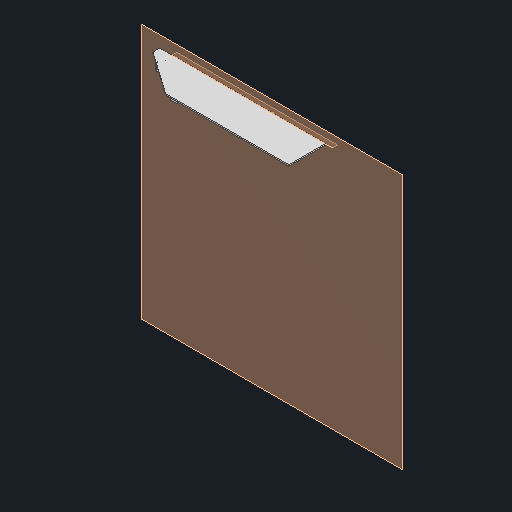
# Autodesk Inventor part: right_side
Saved by Autodesk Inventor 2023 (Build 270158000, 158)
## iProperties
Created: 2024-05-19
Part Number: right_side
Material: Generic
Document SubType Name: Modeling
Designer: szymo
Density: 1 g/cm^3
Appearance: Default
Mass: 4.02235 g
Surface Area: 72.4385 cm^2
Volume: 4.02235 cm^3
Author: szymo
Autodesk Inventor part; units mm, degrees
ref_plane "YZ Plane" through (0, 0, 0) normal (1, 0, 0) x (0, 1, 0)
ref_plane "XZ Plane" through (0, 0, 0) normal (0, 1, 0) x (-1, 0, 0)
ref_plane "XY Plane" through (0, 0, 0) normal (0, 0, 1) x (1, 0, 0)
ref_plane "Work Plane1" through (41, 89, -3.5) normal (0, 1, 0) x (-1, 0, 0)
sketch "Sketch1" plane through (41, 89, -3.5) normal (0, 1, 0) x (-1, 0, 0)
  arc A0 (0, 27.0092) -> (4.4908, 31.5) centre (3, 28.5) ccw projected
  line L0 (0, 3.5) -> (0, 27.0092) projected
  line L1 (0, 3.5) -> (99.4519, 3.5) projected
  line L2 (99.4519, 3.5) -> (97.9046, 17.0805) projected
  line L3 (97.9046, 17.0805) -> (86.1669, 8.8617) projected
  line L4 (85.0198, 8.5) -> (76.1137, 8.5) projected
  line L5 (74.9666, 12.1383) -> (92.1507, 24.1708) projected
  line L6 (94.445, 24.1708) -> (98.8981, 21.0527) projected
  line L7 (99.5829, 18.612) -> (109.4208, 19.7329) projected
  line L8 (109.4208, 19.7329) -> (111.1189, 4.8293) projected
  line L9 (111.1189, 4.8293) -> (99.4519, 3.5) projected
  line L10 (99.4519, 3.5) -> (127, 3.5) projected
  line L11 (127, 3.5) -> (127, 8.7002) projected
  line L12 (127, 8.7002) -> (123.75, 8.7002) projected
  line L13 (123.75, 8.7002) -> (120.5, 8.7002) projected
  arc A1 (116.1068, 16.3277) -> (120.5, 8.7002) centre (127.9773, 18.0858) ccw projected
  line L14 (116.1068, 16.3277) -> (94.4385, 31.5) projected
  line L15 (94.4385, 31.5) -> (27.4908, 31.5) projected
  arc A2 (24.5092, 31.5) -> (27.4908, 31.5) centre (26, 28.5) ccw projected
  line L16 (24.5092, 31.5) -> (4.4908, 31.5) projected
  circle A3 centre (15.5, 17.5) radius 5 projected
  arc A4 (6.5587, 12.2463) -> (10.9717, 8.1704) centre (15.5, 17.5) ccw projected
  arc A5 (7.2428, 14.3769) -> (6.5587, 12.2463) centre (7.852, 13.0062) ccw projected
  line L17 (7.2428, 14.3769) -> (8.2553, 14.827) projected
  arc A6 (10.1455, 14.2369) -> (8.2553, 14.827) centre (8.8646, 13.4563) ccw projected
  arc A7 (10.1455, 14.2369) -> (12.6717, 11.9036) centre (15.5, 17.5) ccw projected
  arc A8 (13.4098, 10.0662) -> (12.6717, 11.9036) centre (11.9951, 10.5649) ccw projected
  line L18 (13.4098, 10.0662) -> (13.0414, 9.0211) projected
  arc A9 (10.9717, 8.1704) -> (13.0414, 9.0211) centre (11.6267, 9.5198) ccw projected
  arc A10 (20.0283, 26.8296) -> (17.9586, 25.9789) centre (19.3733, 25.4802) ccw projected
  arc A11 (24.4413, 22.7537) -> (20.0283, 26.8296) centre (15.5, 17.5) ccw projected
  arc A12 (23.7572, 20.6231) -> (24.4413, 22.7537) centre (23.148, 21.9938) ccw projected
  line L19 (23.7572, 20.6231) -> (22.7447, 20.173) projected
  arc A13 (20.8545, 20.7631) -> (22.7447, 20.173) centre (22.1354, 21.5437) ccw projected
  arc A14 (20.8545, 20.7631) -> (18.3283, 23.0964) centre (15.5, 17.5) ccw projected
  arc A15 (17.5902, 24.9338) -> (18.3283, 23.0964) centre (19.0049, 24.4351) ccw projected
  line L20 (17.5902, 24.9338) -> (17.9586, 25.9789) projected
  arc A16 (6.5587, 22.7537) -> (7.2428, 20.6231) centre (7.852, 21.9938) ccw projected
  arc A17 (10.9717, 26.8296) -> (6.5587, 22.7537) centre (15.5, 17.5) ccw projected
  arc A18 (13.0414, 25.9789) -> (10.9717, 26.8296) centre (11.6267, 25.4802) ccw projected
  line L21 (13.0414, 25.9789) -> (13.4098, 24.9338) projected
  arc A19 (12.6717, 23.0964) -> (13.4098, 24.9338) centre (11.9951, 24.4351) ccw projected
  arc A20 (8.2553, 20.173) -> (10.1455, 20.7631) centre (8.8646, 21.5437) ccw projected
  line L22 (8.2553, 20.173) -> (7.2428, 20.6231) projected
  arc A21 (20.0283, 8.1704) -> (24.4413, 12.2463) centre (15.5, 17.5) ccw projected
  arc A22 (17.9586, 9.0211) -> (20.0283, 8.1704) centre (19.3733, 9.5198) ccw projected
  line L23 (17.9586, 9.0211) -> (17.5902, 10.0662) projected
  arc A23 (18.3283, 11.9036) -> (17.5902, 10.0662) centre (19.0049, 10.5649) ccw projected
  arc A24 (18.3283, 11.9036) -> (20.8545, 14.2369) centre (15.5, 17.5) ccw projected
  arc A25 (22.7447, 14.827) -> (20.8545, 14.2369) centre (22.1354, 13.4563) ccw projected
  line L24 (22.7447, 14.827) -> (23.7572, 14.3769) projected
  arc A26 (24.4413, 12.2463) -> (23.7572, 14.3769) centre (23.148, 13.0062) ccw projected
  line L25 (60.4227, 8.5) -> (45.5604, 8.5) projected
  line L26 (44.4133, 12.1383) -> (64.4073, 26.1383) projected
  line L27 (65.5545, 26.5) -> (80.4168, 26.5) projected
  line L28 (81.5639, 22.8617) -> (61.5699, 8.8617) projected
  line L29 (30.5, 12.342) -> (30.5, 26.5) projected
  line L30 (32.5, 28.5) -> (52.7198, 28.5) projected
  line L31 (53.8669, 24.8617) -> (33.6472, 10.7037) projected
  line L32 (0, 3.5) -> (94.4385, 3.5)
  line L33 (94.4385, 3.5) -> (94.4385, 31.5)
  line L34 (94.4385, 31.5) -> (0, 31.5)
  line L35 (0, 31.5) -> (0, 3.5)
  line L36 (94.4385, 31.5) -> (127, 8.7002)
  line L37 (127, 8.7002) -> (127, 3.5)
  line L38 (127, 3.5) -> (94.4385, 3.5)
  arc A27 (12.6717, 23.0964) -> (10.1455, 20.7631) centre (15.5, 17.5) ccw projected
  arc A28 (85.0198, 8.5) -> (86.1669, 8.8617) centre (85.0198, 10.5) ccw projected
  arc A29 (74.9666, 12.1383) -> (76.1137, 8.5) centre (76.1137, 10.5) ccw projected
  arc A30 (94.445, 24.1708) -> (92.1507, 24.1708) centre (93.2979, 22.5325) ccw projected
  arc A31 (99.5829, 18.612) -> (98.8981, 21.0527) centre (97.7509, 19.4144) ccw projected
  circle A32 centre (15.5, 25.5) radius 1.8 projected
  circle A33 centre (15.5, 9.5) radius 1.8 projected
  arc A34 (44.4133, 12.1383) -> (45.5604, 8.5) centre (45.5604, 10.5) ccw projected
  arc A35 (65.5545, 26.5) -> (64.4073, 26.1383) centre (65.5545, 24.5) ccw projected
  arc A36 (81.5639, 22.8617) -> (80.4168, 26.5) centre (80.4168, 24.5) ccw projected
  arc A37 (60.4227, 8.5) -> (61.5699, 8.8617) centre (60.4227, 10.5) ccw projected
  arc A38 (32.5, 28.5) -> (30.5, 26.5) centre (32.5, 26.5) ccw projected
  arc A39 (53.8669, 24.8617) -> (52.7198, 28.5) centre (52.7198, 26.5) ccw projected
  arc A40 (30.5, 12.342) -> (33.6472, 10.7037) centre (32.5, 12.342) ccw projected
  point P0 (41, 3.5)
  point P1 (27.4908, 31.5)
  point P2 (24.5092, 31.5)
  point P3 (4.4908, 31.5)
  point P4 (0, 27.0092)
  constraints: 14 end point, 3 equal length, 2 perpendicular, 1 horizontal
extrude "Extrusion1" add sketch "Sketch1" against normal blind 1 contours L35 L34 A0 | A0 L16 A2 L15 L33 A30 L5 A29 L4 A28 L3 L1 L0 | L34 A2 | L33 L3 L2 L1 | L2 L3 L33 A30 L6 A31 L7 L8 L9 | L9 L8 L7 A31 L6 A30 L33 L14 A1 L13 L12 L11 L10 | L3 A28 L4 A29 L5 A30 L33 | L36 L12 L13 A1 | A3 | A5 L17 A6 A7 A8 L18 A9 A4 | A11 A12 L19 A13 A14 A15 L20 A10 | A17 A18 L21 A19 A27 A20 L22 A16 | A22 L23 A23 A24 A25 L24 A26 A21 | L25 A34 L26 A35 L27 A36 L28 A37 | L29 A38 L30 A39 L31 A40 | A32 | A33
sketch "Sketch2" plane through (41, 88, -3.5) normal (0, -1, 0) x (1, 0, 0)
  point P0 (-41, 3.5)
sketch "Sketch3" plane through (41, 88, -3.5) normal (0, -1, 0) x (1, 0, 0)
  line L0 (-127, 3.5) -> (0, 3.5) projected
  line L1 (0, 3.5) -> (0, 31.5) projected
  line L2 (0, 31.5) -> (-94.4385, 31.5) projected
  line L3 (-94.4385, 31.5) -> (-127, 8.7002) projected
  line L4 (-127, 8.7002) -> (-127, 3.5) projected
  line L5 (-118.25, 3.5) -> (-115.75, 3.5) projected
  line L6 (-118.25, 3.5) -> (-115.75, 3.5)
  line L7 (-115.75, 3.5) -> (-115.75, 7)
  line L8 (-115.75, 7) -> (-118.25, 7)
  line L9 (-118.25, 7) -> (-118.25, 3.5)
  line L10 (-123.5, 5.5) -> (-123.5, 3.5) projected
  line L11 (-121.5, 3.5) -> (-112, 3.5)
  line L12 (-112, 3.5) -> (-112, 19.2033)
  line L13 (-112, 19.2033) -> (-121.5, 19.2033)
  line L14 (-121.5, 19.2033) -> (-121.5, 3.5)
  line L15 (-112.5, 3.5) -> (-126.5, 3.5) projected
  line L16 (-112, 3.5) -> (-128, 3.5) projected
  line L17 (-121.5, 3.5) -> (-112, 3.5)
  line L18 (-112, 3.5) -> (-112, 8.5)
  line L19 (-112, 8.5) -> (-121.5, 8.5)
  line L20 (-121.5, 8.5) -> (-121.5, 3.5)
  point P0 (-41, 3.5)
  dimension "d2" = 3.5
  dimension "d3" = 2
  dimension "d5" = 5
  constraints: 24 end point, 6 parallel, 4 point on line, 3 horizontal, 3 perpendicular, 1 other
  measures "d2" distance of L7.end L6.end
  measures "d3" distance from line of L14 L10.start
  measures "d5" distance between parallel lines of L19 L15
extrude "Extrusion2" add sketch "Sketch3" along normal blind 12 contours L14 L19 L12 L0 L7 L8 L9 | L9 L8 L7 L0
sketch "Sketch4" plane through (41, 88, -3.5) normal (0, -1, 0) x (1, 0, 0)
  line L0 (-121.5, 3.5) -> (-121.5, 8.5) projected
  line L1 (-121.5, 8.5) -> (-112, 8.5) projected
  line L2 (-112, 8.5) -> (-112, 3.5) projected
  line L3 (-112, 3.5) -> (0, 3.5) projected
  line L4 (0, 3.5) -> (0, 31.5) projected
  line L5 (0, 31.5) -> (-94.4385, 31.5) projected
  line L6 (-94.4385, 31.5) -> (-127, 8.7002) projected
  line L7 (-127, 8.7002) -> (-127, 3.5) projected
  line L8 (-127, 3.5) -> (-121.5, 3.5) projected
  line L9 (-121.4366, 12.5958) -> (-117.3408, 15.4636)
  line L10 (-117.3408, 15.4636) -> (-114.4729, 11.3679)
  line L11 (-114.4729, 11.3679) -> (-118.5687, 8.5)
  line L12 (-118.5687, 8.5) -> (-121.4366, 12.5958)
  line L13 (-112, 8.5) -> (-121.5, 8.5) projected
  line L14 (-121.4366, 12.5958) -> (-121.5, 8.5)
  line L15 (-114.4729, 11.3679) -> (-112, 8.5)
  point P0 (-41, 3.5)
  dimension "d8" = 5
  dimension "d9" = 5
  constraints: 12 end point, 3 point on line, 2 parallel, 1 perpendicular
  measures "d8" distance of L9.start L9.end
  measures "d9" distance of L9.end L10.end
extrude "Extrusion3" add sketch "Sketch4" along normal blind 4 contours L14 L12 L1 | L11 L15 L1 | L12 L6 L10 L11
sketch "Sketch5" plane through (-86, 88, 5.2002) normal (-0.5735764, 0, 0.819152) x (0.819152, 0, 0.5735764)
  line L0 (0, 1) -> (39.7502, 1) projected
  line L1 (0, 1) -> (0, 0) projected
  line L2 (6.7917, 0) -> (0, 0) projected
  line L3 (6.7917, 0) -> (6.7917, -4) projected
  line L4 (11.7917, -4) -> (6.7917, -4) projected
  line L5 (11.7917, 0) -> (11.7917, -4) projected
  line L6 (39.7502, 0) -> (11.7917, 0) projected
  line L7 (39.7502, 1) -> (39.7502, 0) projected
  line L8 (6.7917, -4) -> (11.7917, -4)
  line L9 (11.7917, -4) -> (11.7917, 1)
  line L10 (11.7917, 1) -> (6.7917, 1)
  line L11 (6.7917, 1) -> (6.7917, -4)
  line L12 (11.7917, -4) -> (6.7917, 1)
  line L13 (6.7917, -4) -> (11.7917, 1)
  line L14 (9.3046, 0) -> (9.3046, -12) projected
  point P0 (67.4644, -88)
  point P1 (9.3046, -1.4871)
  constraints: 12 end point, 3 point on line, 2 parallel, 2 perpendicular, 1 horizontal
hole "Hole1" at (-78.3781, 86.5129, 10.5371) direction (0.5735764, 0, -0.819152) diameter 4 depth 5.5 counterbore diameter 4.6 counterbore depth 1
ref_plane "Work Plane2" through (0, 0, 0) normal (0, 0, 1) x (1, 0, 0)
sketch "Sketch6" plane through (0, 0, 0) normal (0, 0, 1) x (1, 0, 0)
  ellipse E0 centre (-78.3781, 86.5129) end of major axis (-78.3781, 84.2129) minor radius 1.884 projected
  line L0 (-86, 89) -> (-53.4385, 89) projected
  line L1 (-86, 89) -> (-86, 88) projected
  line L2 (-80.4366, 88) -> (-86, 88) projected
  line L3 (-80.4366, 88) -> (-80.4366, 84) projected
  line L4 (-76.3408, 84) -> (-80.4366, 84) projected
  line L5 (-76.3408, 88) -> (-76.3408, 84) projected
  line L6 (-53.4385, 88) -> (-76.3408, 88) projected
  line L7 (-53.4385, 89) -> (-53.4385, 88) projected
  line L8 (-73.4729, 88) -> (-71, 88) projected
  line L9 (-73.4729, 88) -> (-73.4729, 84) projected
  line L10 (-71, 84) -> (-73.4729, 84) projected
  line L11 (-71, 88) -> (-71, 84) projected
  line L12 (-71, 84) -> (-80.5, 84) projected
  line L13 (-80.5, 84) -> (-80.5, 76) projected
  line L14 (-71, 76) -> (-80.5, 76) projected
  line L15 (-71, 84) -> (-71, 76) projected
  line L16 (-71, 88) -> (-71, 76) projected
  line L17 (-71, 88) -> (-64, 88)
  line L18 (-64, 88) -> (-64, 81)
  line L19 (-64, 81) -> (-71, 81)
  line L20 (-71, 81) -> (-71, 88)
  point P0 (0, 0)
  dimension "d19" = 7
  dimension "d20" = 7
  constraints: 8 end point, 2 parallel, 1 horizontal, 1 perpendicular, 1 other
  measures "d19" distance of L18.end L19.end
  measures "d20" distance of L17.end L18.end
extrude "Extrusion4" add sketch "Sketch6" along normal up to surface (5 mm away) contours L18 L19 L15 L11 L6
sketch "Sketch7" plane through (-80.5, 76, 5) normal (0, 0, 1) x (1, 0, 0)
  line L0 (9.5, 8) -> (0, 8) projected
  line L1 (0, 8) -> (0, 0) projected
  line L2 (9.5, 0) -> (0, 0) projected
  line L3 (9.5, 5) -> (9.5, 0) projected
  line L4 (16.5, 5) -> (9.5, 5) projected
  line L5 (16.5, 12) -> (16.5, 5) projected
  line L6 (9.5, 12) -> (16.5, 12) projected
  line L7 (9.5, 12) -> (9.5, 8) projected
  line L8 (16.5, 5) -> (9.5, 12)
  point P0 (80.5, -76)
  point P1 (13, 8.5)
  constraints: 2 end point, 1 midpoint
hole "Hole2" at (-67.5, 84.5, 5) direction (0, 0, -1) diameter 3.6 end through all countersink diameter 6.5 countersink angle 90 clearance for "Countersunk Flat Head Screw ISO 2009/7046" size "M3" standard "ISO"
ref_plane "Work Plane3" through (0, 0, 0) normal (0, 0, 1) x (1, 0, 0)
sketch "Sketch9" plane through (-71, 81, 0) normal (0, -1, 0) x (1, 0, 0)
  line L0 (7, 5) -> (0, 5) projected
  line L1 (0, 0) -> (0, 5) projected
  line L2 (0, 0) -> (7, 0) projected
  line L3 (7, 0) -> (7, 5) projected
  line L4 (0, 5) -> (7, 5) projected
  line L5 (7, 5) -> (7, 0) projected
  line L6 (7, 0) -> (112, 0) projected
  line L7 (112, 0) -> (112, 28) projected
  line L8 (112, 28) -> (17.5615, 28) projected
  line L9 (17.5615, 28) -> (-5.3408, 11.9636) projected
  line L10 (-5.3408, 11.9636) -> (-2.4729, 7.8679) projected
  line L11 (-2.4729, 7.8679) -> (0, 5) projected
  line L12 (8.4872, 5.8762) -> (8.063, 2.1531) projected
  ellipse E0 centre (35.1181, -1.499) end of major axis (68.222, -5.1272) minor radius 1.1914 (12.7569, 1.8325) -> (8.063, 2.1531) ccw projected
  line L13 (13.157, 5.3441) -> (12.7569, 1.8325) projected
  line L14 (8.4872, 5.8762) -> (13.157, 5.3441) projected
  line L15 (14.0374, 13.0711) -> (13.6373, 9.5595) projected
  ellipse E1 centre (36.5749, 11.287) end of major axis (3.5033, 15.1985) minor radius 1.1914 (9.3917, 13.8146) -> (14.0374, 13.0711) ccw projected
  line L16 (9.3917, 13.8146) -> (8.9675, 10.0915) projected
  line L17 (8.9675, 10.0915) -> (13.6373, 9.5595) projected
  line L18 (8.5623, 9.1853) -> (13.5302, 8.6192)
  line L19 (8.2963, 6.8504) -> (13.2641, 6.2843)
  line L20 (7, 0) -> (0, 0)
  line L21 (0, 0) -> (0, 5)
  line L22 (0, 5) -> (7, 5)
  line L23 (7, 5) -> (7, 0)
  point P0 (71, 0)
  constraints: 12 end point, 2 parallel, 1 horizontal, 1 perpendicular, 8 other
extrude "Extrusion5" add sketch "Sketch9" along normal blind 12 contours L3 L2 L1 L0
sketch "Sketch10" plane through (-71, 69, 0) normal (0, -1, 0) x (1, 0, 0)
  line L0 (7, 5) -> (0, 5) projected
  line L1 (0, 5) -> (0, 0) projected
  line L2 (0, 0) -> (7, 0) projected
  line L3 (7, 0) -> (7, 5) projected
  line L4 (4.2431, 13.9877) -> (8.8553, 13.6247) projected
  ellipse E0 centre (9.2065, 13.1962) end of major axis (9.0904, 12.4558) minor radius 0.4749 (8.8553, 13.6247) -> (8.7306, 13.2204) ccw projected
  line L5 (8.7306, 13.2204) -> (7.5526, 2.8808) projected
  ellipse E1 centre (8.0217, 2.7973) end of major axis (7.9684, 2.0497) minor radius 0.4749 (7.5526, 2.8808) -> (7.5831, 2.4588) ccw projected
  line L6 (7.5831, 2.4588) -> (3.0075, 3.1426) projected
  line L7 (3.0075, 3.1426) -> (3.0079, 3.1457) projected
  line L8 (3.0079, 3.1457) -> (4.2428, 13.9845) projected
  line L9 (4.2428, 13.9845) -> (4.2431, 13.9877) projected
  line L10 (8.5623, 9.1853) -> (13.5302, 8.6192)
  line L11 (8.2963, 6.8504) -> (13.2641, 6.2843)
  line L12 (8.5623, 9.1853) -> (8.2963, 6.8504)
  line L13 (8.2963, 6.8504) -> (3.3284, 7.4164)
  line L14 (3.3284, 7.4164) -> (3.5944, 9.7513)
  line L15 (3.5944, 9.7513) -> (8.5623, 9.1853)
  line L16 (3.7076, 10.7448) -> (8.6755, 10.1788)
  line L17 (8.6755, 10.1788) -> (8.1831, 5.8568)
  line L18 (8.1831, 5.8568) -> (3.2152, 6.4228)
  line L19 (3.2152, 6.4228) -> (3.7076, 10.7448)
  line L20 (7, 5) -> (7, 0) projected
  line L21 (8.1831, 5.8568) -> (7, 0)
  line L22 (3.7076, 10.7448) -> (0, 5)
  point P0 (71, 0)
  point P1 (8.2963, 6.8504)
  point P2 (8.5623, 9.1853)
  dimension "d32" = 5
  dimension "d33" = 1
  dimension "d34" = 1
  constraints: 24 end point, 5 parallel, 2 collinear, 2 perpendicular, 8 other
  measures "d32" distance of L11.start L13.end
  measures "d33" distance between parallel lines of L16 L15
  measures "d34" distance between parallel lines of L13 L18
extrude "Extrusion6" add sketch "Sketch10" against normal blind 5 contours L3 L6 L7 L8 L0 | L0 L8 L18 L5 E1 L21 L6 L3 | L8 L7 L6 L3 L2 L1 L0 | L0 L22 L19 L14 L18 L8 | L6 L21 L3 | L18 L19 L13 L8 | L8 L13 L5 L18 | L16 L8 L15 L19 | L13 L14 L15 L8 | L8 L15 L5 L13 | L18 L21 E1 L5 | L5 L13 L17 L18 | L16 L5 L15 L8 | L5 L15 L12 L13 | L16 L17 L15 L5
sketch "Sketch11" plane through (-62.8169, 69, 5.8568) normal (0.9935719, 0, -0.1132032) x (-0.1132032, 0, -0.9935719)
  circle A0 centre (-2.175, 1.6151) radius 1.175 projected
  point P0 (-1.2919, -69)
  constraints: 1 coincident
hole "Hole3" at (-62.5707, 70.6151, 8.0178) direction (-0.9935719, 0, 0.1132032) diameter 1.6 end through all counterbore diameter 4.4 counterbore depth 0
chamfer "Chamfer1" distance 0.5 angle 45 1 edges at (-62.4801, 70.6151, 8.8127)
body "Solid1"
